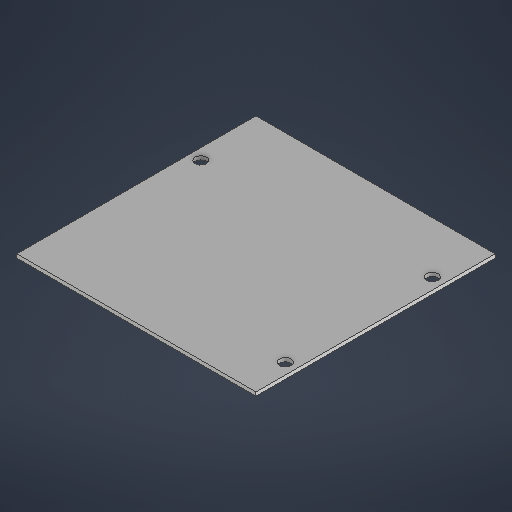
# Autodesk Inventor part: PCB
Saved by Autodesk Inventor 2026 (Build 300175000, 175)
## iProperties
Created: 2025-04-26
Part Number: PCB
Material: Generic
Document SubType Name: Modeling
Designer: isan
Density: 1 g/cm^3
Appearance: Default
Author: isan
Autodesk Inventor part; units mm, degrees
ref_plane "YZ Plane" through (0, 0, 0) normal (1, 0, 0) x (0, 1, 0)
ref_plane "XZ Plane" through (0, 0, 0) normal (0, 1, 0) x (-1, 0, 0)
ref_plane "XY Plane" through (0, 0, 0) normal (0, 0, 1) x (1, 0, 0)
sketch "Sketch1" plane through (0, 0, 0) normal (0, 0, 1) x (1, 0, 0)
  line L0 (-32.6, -32.6) -> (32.6, -32.6)
  line L1 (32.6, -32.6) -> (32.6, 32.6)
  line L2 (32.6, 32.6) -> (-32.6, 32.6)
  line L3 (-32.6, 32.6) -> (-32.6, -32.6)
  line L4 (-32.6, -32.6) -> (32.6, 32.6) construction
  line L5 (32.6, -32.6) -> (-32.6, 32.6) construction
  point P0 (0, 0)
  dimension "d0" = 65.2
  dimension "d1" = 65.2
  constraints: 12 end point, 2 midpoint, 2 parallel, 1 horizontal, 1 perpendicular
  measures "d0" distance of L1.end L2.end
  measures "d1" distance of L0.end L1.end
extrude "Extrusion1" add sketch "Sketch1" along normal blind 1
sketch "Sketch2" plane through (0, 0, 1) normal (0, 0, 1) x (1, 0, 0)
  circle A0 centre (-29.6, 14.557) radius 1.575
  circle A1 centre (29.525, 18.595) radius 1.575
  circle A2 centre (29.583, -21.6) radius 1.575
  line L0 (-32.6, 32.6) -> (-32.6, -32.6) projected
  line L1 (32.6, 32.6) -> (-32.6, 32.6) projected
  line L2 (32.6, -32.6) -> (32.6, 32.6) projected
  line L3 (-32.6, -32.6) -> (32.6, -32.6) projected
  point P0 (0, 0)
  dimension "d4" = 3
  dimension "d5" = 18.043
  dimension "d6" = 3.075
  dimension "d7" = 14.005
  dimension "d8" = 11
  dimension "d9" = 3.017
  dimension "d10" = 3.15
  dimension "d11" = 3.15
  dimension "d12" = 3.15
  constraints: 3 centre point
  measures "d4" distance from line of L0 A0.centre
  measures "d5" distance from line of L1 A0.centre
  measures "d6" distance from line of L2 A1.centre
  measures "d7" distance from line of L1 A1.centre
  measures "d8" distance from line of L3 A2.centre
  measures "d9" distance from line of L2 A2.centre
  measures "d10" diameter of A0
  measures "d11" diameter of A1
  measures "d12" diameter of A2
extrude "Extrusion2" cut sketch "Sketch2" against normal blind 1 contours A0 | A1 | A2
body "Solid1"
